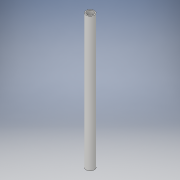
# Autodesk Inventor part: Axle_2_KFuchs
Saved by Autodesk Inventor 2019 (Build 230136000, 136)
## iProperties
Created: 2019-05-10
Part Number: Axle_2_KFuchs
Material: Generic
Document SubType Name: Modeling
Designer: kyle.fuchs
Density: 1 g/cm^3
Appearance: Default
Author: kyle.fuchs
Autodesk Inventor part; units mm, degrees
ref_plane "YZ Plane" through (0, 0, 0) normal (1, 0, 0) x (0, 1, 0)
ref_plane "XZ Plane" through (0, 0, 0) normal (0, 1, 0) x (-1, 0, 0)
sketch "Sketch1" plane through (0, 0, 0) normal (0, 1, 0) x (-1, 0, 0)
  circle A0 centre (0, 0) radius 12.7
  circle A1 centre (0, 0) radius 9.652
  dimension "d0" = 25.4
  dimension "d1" = 19.304
  constraints: 2 centre point, 2 coincident
  measures "d0" diameter of A0
  measures "d1" diameter of A1
extrude "Extrusion1" add sketch "Sketch1" along normal mid plane 406.4
sketch "Sketch2" plane through (0, 203.2, 0) normal (0, 1, 0) x (1, 0, 0)
  circle A0 centre (0, 0) radius 12.7 projected
  line L0 (-13.8417, 2.54) -> (-12.4434, 2.54)
  line L1 (-13.8417, -2.54) -> (-12.4434, -2.54)
  line L2 (-13.8417, -2.54) -> (-13.8417, 2.54)
  constraints: 6 end point, 2 point on circle
extrude "Extrusion2" add sketch "Sketch2" against normal blind 200.025 contours A0 L1 L2 L0
sketch "Sketch3" plane through (0, 203.2, 0) normal (0, 1, 0) x (1, 0, 0)
  circle A0 centre (0, 0) radius 12.7 projected
  line L0 (-12.4434, -2.54) -> (-13.8417, -2.54) projected
  line L1 (-12.4434, -2.54) -> (-13.8417, -2.54)
  line L2 (-13.8417, 2.54) -> (-12.4434, 2.54) projected
  line L3 (-13.8417, -2.54) -> (-13.8417, 2.54)
  line L4 (-13.8417, 2.54) -> (-12.4434, 2.54)
  constraints: 6 end point, 2 perpendicular, 1 horizontal, 1 point on circle
extrude "Extrusion3" cut sketch "Sketch3" against normal blind 6.35 contours A0 L0 L3 L2
ref_plane "Work Plane2" through (0, 0, 0) normal (0, -1, 0) x (1, 0, 0)
sketch "Sketch7" plane through (0, 0, 0) normal (0, -1, 0) x (1, 0, 0)
  line L0 (-13.8417, 2.5539) -> (-13.8417, -2.54) projected
  line L1 (-13.8417, 0.0069) -> (-13.8417, -3.1681)
  line L2 (-13.8417, 0.0069) -> (-13.8417, 3.1819)
  circle A0 centre (0, 0) radius 12.7 projected
  line L3 (-13.8417, -3.1681) -> (-12.2949, -3.1681)
  line L4 (-12.2949, -3.1681) -> (-12.2949, 3.1819)
  line L5 (-12.2949, 3.1819) -> (-13.8417, 3.1819)
  line L6 (-13.8417, 3.1819) -> (-13.8417, -3.1681)
  dimension "d14" = 3.175
  dimension "d15" = 3.175
  constraints: 12 end point, 2 parallel, 1 collinear, 1 horizontal, 1 midpoint, 1 perpendicular, 1 point on line, 2 other
  measures "d14" distance of L1.start L1.end
  measures "d15" distance of L1.start L2.end
extrude "Extrusion5" add sketch "Sketch7" along normal blind 3.175 contours L2 L5 A0 L3 L1 L0 | L4 L3 A0 picked at (-12.4147, 0.3631)
body "Solid1"
